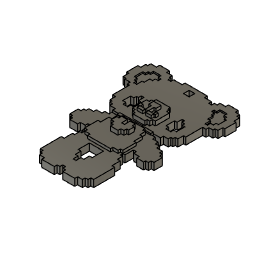
urs tema 1 varianta finala (Autodesk Fusion 360 design; units mm, degrees)
Autodesk Fusion 360 part; units mm, degrees
sketch "bear" plane through (0, 0, 0) normal (0, 0, 1) x (1, 0, 0)
  line L0 (-14, 45) -> (-7, 45)
  line L1 (-7, 45) -> (-7, 43)
  line L2 (-7, 43) -> (-3, 43)
  line L3 (-3, 43) -> (-3, 41)
  line L4 (-3, 41) -> (-2, 41)
  line L5 (-2, 41) -> (-2, 39)
  line L6 (-2, 39) -> (0, 39)
  line L7 (0, 39) -> (0, 41)
  line L8 (0, 41) -> (6, 41)
  line L9 (6, 41) -> (6, 43)
  line L10 (6, 43) -> (22, 43)
  line L11 (22, 43) -> (22, 41)
  line L12 (22, 41) -> (27, 41)
  line L13 (27, 41) -> (27, 39)
  line L14 (27, 39) -> (29, 39)
  line L15 (29, 39) -> (29, 41)
  line L16 (29, 41) -> (31, 41)
  line L17 (31, 41) -> (31, 43)
  line L18 (35, 43) -> (35, 45)
  line L19 (35, 45) -> (42, 45)
  line L20 (42, 45) -> (42, 43)
  line L21 (31, 43) -> (35, 43)
  line L22 (45, 43) -> (42, 43)
  line L23 (45, 43) -> (45, 41)
  line L24 (45, 41) -> (47, 41)
  line L25 (47, 41) -> (47, 37)
  line L26 (47, 37) -> (48.4791, 37)
  line L27 (48.4791, 37) -> (48.4791, 29)
  line L28 (48.4791, 29) -> (47, 29)
  line L29 (47, 29) -> (47, 25.5234)
  line L30 (47, 25.5234) -> (45, 25.5234)
  line L31 (45, 25.5234) -> (45, 24)
  line L32 (45, 24) -> (42, 24)
  line L33 (42, 24) -> (42, 22)
  line L34 (42, 22) -> (39.6461, 22)
  line L35 (39.6461, 22) -> (39.6461, 10)
  line L36 (39.6461, 10) -> (38, 10)
  line L37 (38, 10) -> (38, 6)
  line L38 (38, 6) -> (36, 6)
  line L39 (36, 6) -> (36, 4.4339)
  line L40 (36, 4.4339) -> (34.4937, 4.4339)
  line L41 (34.4937, 4.4339) -> (34.4937, 2.6047)
  line L42 (34.4937, 2.6047) -> (31.118, 2.6047)
  line L43 (31.118, 2.6047) -> (31.118, 0.4845)
  line L44 (31.118, 0.4845) -> (26, 0.4845)
  line L45 (26, 0.4845) -> (26, -1)
  line L46 (26, -1) -> (29, -1)
  line L47 (29, -1) -> (29, -3)
  line L48 (29, -3) -> (33, -3)
  line L49 (33, -3) -> (33, -5)
  line L50 (33, -5) -> (36, -5)
  line L51 (36, -5) -> (36, -7)
  line L52 (36, -7) -> (40, -7)
  line L53 (40, -7) -> (40, -9)
  line L54 (40, -9) -> (42, -9)
  line L55 (42, -9) -> (42, -11)
  line L56 (42, -11) -> (44, -11)
  line L57 (44, -11) -> (44, -17)
  line L58 (44, -17) -> (42, -17)
  line L59 (42, -17) -> (42, -19)
  line L60 (42, -19) -> (40, -19)
  line L61 (40, -19) -> (40, -20.3801)
  line L62 (40, -20.3801) -> (35, -20.3801)
  line L63 (35, -20.3801) -> (35, -18.5424)
  line L64 (35, -18.5424) -> (31, -18.5424)
  line L65 (31, -18.5424) -> (31, -16.5965)
  line L66 (31, -16.5965) -> (29, -16.5965)
  line L67 (29, -16.5965) -> (29, -22.6503)
  line L68 (29, -22.6503) -> (27.3439, -22.6503)
  line L69 (27.3439, -22.6503) -> (27.3439, -24.2966)
  line L70 (27.3439, -24.2966) -> (29, -24.2966)
  line L71 (29, -24.2966) -> (29, -28)
  line L72 (29, -28) -> (31, -28)
  line L73 (31, -28) -> (31, -34)
  line L74 (31, -34) -> (33, -34)
  line L75 (33, -34) -> (33, -49)
  line L76 (33, -49) -> (31, -49)
  line L77 (31, -49) -> (31, -51)
  line L78 (31, -51) -> (29, -51)
  line L79 (29, -51) -> (29, -53)
  line L80 (29, -53) -> (25.5718, -53)
  line L81 (25.5718, -53) -> (25.5718, -55)
  line L82 (25.5718, -55) -> (17, -55)
  line L83 (17, -55) -> (17, -53)
  line L84 (17, -53) -> (15, -53)
  line L85 (15, -53) -> (15, -51)
  line L86 (13, -51) -> (13, -53)
  line L87 (13, -53) -> (11, -53)
  line L88 (11, -53) -> (11, -55)
  line L89 (11, -55) -> (2, -55)
  line L90 (2, -55) -> (2, -53)
  line L91 (2, -53) -> (-1.5352, -53)
  line L92 (-1.5352, -53) -> (-1.5352, -51)
  line L93 (-1.5352, -51) -> (-3, -51)
  line L94 (-3, -51) -> (-3, -49)
  line L95 (-3, -49) -> (-5, -49)
  line L96 (-5, -49) -> (-5, -34)
  line L97 (-5, -34) -> (-3, -34)
  line L98 (-3, -34) -> (-3, -28)
  line L99 (-3, -28) -> (-1.486, -28)
  line L100 (-1.486, -28) -> (-1.486, -24.3526)
  line L101 (-1.486, -24.3526) -> (0, -24.3526)
  line L102 (0, -24.3526) -> (0, -22.7233)
  line L103 (0, -22.7233) -> (-1.486, -22.7233)
  line L104 (-1.486, -22.7233) -> (-1.486, -16.5263)
  line L105 (-1.486, -16.5263) -> (-3.4733, -16.5263)
  line L106 (-3.4733, -16.5263) -> (-3.4733, -18.4756)
  line L107 (-3.4733, -18.4756) -> (-7, -18.4756)
  line L108 (-7, -18.4756) -> (-7, -20.4249)
  line L109 (-7, -20.4249) -> (-12.5396, -20.4249)
  line L110 (-12.5396, -20.4249) -> (-12.5396, -18.4756)
  line L111 (-12.5396, -18.4756) -> (-14, -18.4756)
  line L112 (-14, -18.4756) -> (-14, -17)
  line L113 (-14, -17) -> (-16, -17)
  line L114 (-16, -17) -> (-16, -11)
  line L115 (-16, -11) -> (-14, -11)
  line L116 (-14, -11) -> (-14, -9)
  line L117 (-14, -9) -> (-12.403, -9)
  line L118 (-12.403, -9) -> (-12.403, -7)
  line L119 (-12.403, -7) -> (-9, -7)
  line L120 (-9, -7) -> (-9, -5)
  line L121 (-9, -5) -> (-5, -5)
  line L122 (-5, -5) -> (-5, -3)
  line L123 (-5, -3) -> (-2, -3)
  line L124 (-2, -3) -> (-2, -1)
  line L125 (-2, -1) -> (2, -1)
  line L126 (2, -1) -> (2, 0.5618)
  line L127 (2, 0.5618) -> (-3, 0.5618)
  line L128 (-3, 0.5618) -> (-3, 2.5032)
  line L129 (-3, 2.5032) -> (-7.0312, 2.5032)
  line L130 (-7.0312, 2.5032) -> (-7.0312, 4.4654)
  line L131 (-7.0312, 4.4654) -> (-9, 4.4654)
  line L132 (-9, 4.4654) -> (-9, 6)
  line L133 (-9, 6) -> (-10.3758, 6)
  line L134 (-10.3758, 6) -> (-10.3758, 10)
  line L135 (-10.3758, 10) -> (-12.4717, 10)
  line L136 (-12.4717, 10) -> (-12.4717, 22)
  line L137 (-12.4717, 22) -> (-14, 22)
  line L138 (-14, 22) -> (-14, 24)
  line L139 (-14, 24) -> (-18, 24)
  line L140 (-18, 24) -> (-18, 25)
  line L141 (-18, 25) -> (-20, 25)
  line L142 (-20, 25) -> (-20, 29)
  line L143 (-20, 29) -> (-21.5209, 29)
  line L144 (-21.5209, 29) -> (-21.5209, 37)
  line L145 (-21.5209, 37) -> (-19.4284, 37)
  line L146 (-19.4284, 37) -> (-19.4284, 40.542)
  line L147 (-19.4284, 40.542) -> (-18, 40.542)
  line L148 (-18, 40.542) -> (-18, 42.7271)
  line L149 (-18, 42.7271) -> (-14, 42.7271)
  line L150 (-14, 42.7271) -> (-14, 45)
  line L151 (15, -51) -> (14, -51)
  line L152 (14, -51) -> (14, -43.4733)
  line L153 (15, -43.4733) -> (15, -40)
  line L154 (15, -40) -> (17, -40)
  line L155 (17, -40) -> (17, -36)
  line L156 (17, -36) -> (19, -36)
  line L157 (19, -36) -> (19, -28)
  line L158 (19, -28) -> (9, -28)
  line L159 (9, -28) -> (9, -36)
  line L160 (9, -36) -> (11, -36)
  line L161 (11, -36) -> (11, -40)
  line L162 (11, -40) -> (13, -40)
  line L163 (13, -40) -> (13, -43.5179)
  line L164 (13, -51) -> (14, -51)
  line L165 (13, -43.5179) -> (14, -43.4733)
  line L166 (15, -43.4733) -> (14, -43.4733)
  line L167 (9, -5) -> (9, -7)
  line L168 (9, -7) -> (7.3877, -7)
  line L169 (7.3877, -7) -> (7.3877, -11)
  line L170 (7.3877, -11) -> (9.335, -11)
  line L171 (9.335, -11) -> (9.335, -13)
  line L172 (9.335, -13) -> (11, -13)
  line L173 (11, -13) -> (11, -15)
  line L174 (11, -15) -> (16.4316, -15)
  line L175 (16.4316, -15) -> (16.4316, -13)
  line L176 (16.4316, -13) -> (18.5952, -13)
  line L177 (18.5952, -13) -> (18.5952, -11)
  line L178 (18.5952, -11) -> (20, -11)
  line L179 (20, -11) -> (20, -7)
  line L180 (20, -7) -> (18.5952, -7)
  line L181 (18.5952, -7) -> (18.5952, -5)
  line L182 (18.5952, -5) -> (15, -5)
  line L183 (15, -5) -> (15, -7)
  line L184 (15, -7) -> (15, -9)
  line L185 (15, -9) -> (13, -9)
  line L186 (13, -9) -> (13, -7)
  line L187 (13, -7) -> (13, -5)
  line L188 (13, -5) -> (9, -5)
  line L189 (29.0368, 19.5758) -> (27.4228, 19.5758)
  line L190 (27.4228, 19.5758) -> (27.4228, 16)
  line L191 (27.4228, 16) -> (25.6136, 16)
  line L192 (25.6136, 16) -> (25.6136, 10)
  line L193 (25.6136, 10) -> (27.4228, 10)
  line L194 (27.4228, 10) -> (27.4228, 8)
  line L195 (27.4228, 8) -> (31, 8)
  line L196 (31, 8) -> (31, 10)
  line L197 (31, 10) -> (33, 10)
  line L198 (33, 10) -> (33, 16)
  line L199 (33, 16) -> (31, 16)
  line L200 (31, 16) -> (31, 17.6991)
  line L201 (31, 17.6991) -> (29.0368, 17.6991)
  line L202 (29.0368, 17.6991) -> (29.0368, 19.5758)
  line L203 (-1.6244, 19.559) -> (-1.6244, 17.5769)
  line L204 (-1.6244, 17.5769) -> (-3, 17.5769)
  line L205 (-3, 17.5769) -> (-3, 15.6458)
  line L206 (-3, 15.6458) -> (-5.3027, 15.6458)
  line L207 (-5.3027, 15.6458) -> (-5.3027, 10)
  line L208 (-5.3027, 10) -> (-3, 10)
  line L209 (-3, 10) -> (-3, 8)
  line L210 (-3, 8) -> (0.276, 8)
  line L211 (0.276, 8) -> (0.276, 10)
  line L212 (0.276, 10) -> (2, 10)
  line L213 (2, 10) -> (2, 15.6458)
  line L214 (2, 15.6458) -> (0.276, 15.6458)
  line L215 (0.276, 15.6458) -> (0.276, 19.559)
  line L216 (0.276, 19.559) -> (-1.6244, 19.559)
  line L217 (8.9896, 19.5636) -> (19, 19.5636)
  line L218 (19, 19.5636) -> (19, 18)
  line L219 (19, 18) -> (20, 18)
  line L220 (20, 18) -> (20, 16)
  line L221 (20, 16) -> (22, 16)
  line L222 (22, 16) -> (22, 6)
  line L223 (22, 6) -> (20, 6)
  line L224 (20, 6) -> (20, 4)
  line L225 (20, 4) -> (19, 4)
  line L226 (19, 4) -> (18, 4)
  line L227 (18, 4) -> (18, 2.4642)
  line L228 (18, 2.4642) -> (9.4555, 2.4642)
  line L229 (9.4555, 2.4642) -> (9.4555, 4)
  line L230 (9.4555, 4) -> (7.5988, 4)
  line L231 (7.5988, 4) -> (7.5988, 6)
  line L232 (7.5988, 6) -> (5.6945, 6)
  line L233 (5.6945, 6) -> (5.6945, 16)
  line L234 (5.6945, 16) -> (7.5988, 16)
  line L235 (7.5988, 16) -> (7.5988, 17.676)
  line L236 (7.5988, 17.676) -> (9, 17.676)
  line L237 (9, 17.676) -> (8.9896, 19.5636)
  line L238 (16.384, 15.6246) -> (16.384, 12)
  line L239 (16.384, 12) -> (15, 12)
  line L240 (15, 12) -> (15, 8)
  line L241 (15, 8) -> (18.5099, 8)
  line L242 (18.5099, 8) -> (18.5099, 10)
  line L243 (18.5099, 10) -> (20, 10)
  line L244 (20, 10) -> (20, 8)
  line L245 (20, 8) -> (19, 8)
  line L246 (19, 8) -> (19, 6)
  line L247 (19, 6) -> (15, 6)
  line L248 (15, 6) -> (15, 7.7223)
  line L249 (15, 7.7223) -> (13, 7.7223)
  line L250 (13, 7.7223) -> (13, 6)
  line L251 (13, 6) -> (9, 6)
  line L252 (9, 6) -> (9, 8)
  line L253 (9, 8) -> (7.4709, 8)
  line L254 (7.4709, 8) -> (7.4709, 10)
  line L255 (7.4709, 10) -> (9.3025, 10)
  line L256 (9.3025, 10) -> (9.3025, 8)
  line L257 (9.3025, 8) -> (13, 8)
  line L258 (13, 8) -> (13, 12.1247)
  line L259 (13, 12.1247) -> (11.1512, 12.1247)
  line L260 (11.1512, 12.1247) -> (11.1512, 15.6246)
  line L261 (11.1512, 15.6246) -> (16.384, 15.6246)
  line L262 (33.0271, 36.6906) -> (35, 36.6906)
  line L263 (35, 36.6906) -> (35, 39)
  line L264 (35, 39) -> (40, 39)
  line L265 (40, 39) -> (40, 36.6906)
  line L266 (40, 36.6906) -> (42, 36.6906)
  line L267 (42, 36.6906) -> (42, 35)
  line L268 (42, 35) -> (43.5849, 35)
  line L269 (43.5849, 35) -> (43.5849, 29.2707)
  line L270 (43.5849, 29.2707) -> (42, 29.2707)
  line L271 (42, 29.2707) -> (42, 27.2792)
  line L272 (42, 27.2792) -> (40, 27.2792)
  line L273 (40, 27.2792) -> (40, 25)
  line L274 (40, 25) -> (38.317, 25)
  line L275 (38.317, 25) -> (38.317, 29)
  line L276 (38.317, 29) -> (36.2934, 29)
  line L277 (36.2934, 29) -> (36.2934, 32.804)
  line L278 (36.2934, 32.804) -> (35, 32.804)
  line L279 (35, 32.804) -> (35, 35)
  line L280 (35, 35) -> (33.0271, 35)
  line L281 (33.0271, 35) -> (33.0271, 36.6906)
  line L282 (-5, 37) -> (-7, 37)
  line L283 (-7, 37) -> (-7, 39)
  line L284 (-7, 39) -> (-12.4235, 39)
  line L285 (-12.4235, 39) -> (-12.4235, 37)
  line L286 (-12.4235, 37) -> (-14, 37)
  line L287 (-14, 37) -> (-14, 35)
  line L288 (-14, 35) -> (-16, 35)
  line L289 (-16, 35) -> (-16, 29)
  line L290 (-16, 29) -> (-14, 29)
  line L291 (-14, 29) -> (-14, 27)
  line L292 (-14, 27) -> (-12.4235, 27)
  line L293 (-12.4235, 27) -> (-12.4235, 25)
  line L294 (-12.4235, 25) -> (-10.3514, 25)
  line L295 (-10.3514, 25) -> (-10.3514, 29)
  line L296 (-10.3514, 29) -> (-9, 29)
  line L297 (-9, 29) -> (-9, 33)
  line L298 (-9, 33) -> (-7, 33)
  line L299 (-7, 33) -> (-7, 35)
  line L300 (-7, 35) -> (-5, 35)
  line L301 (-5, 35) -> (-5, 37)
  line L302 (26, -1) -> (26, -1.349)
  line L303 (26, -1.349) -> (2, -1.349)
  line L304 (2, -1.349) -> (2, -1)
  line L305 (2, 0.5618) -> (26, 0.4845)
  line L306 (5.8111, -1.349) -> (5.8111, -3)
  line L307 (5.8111, -3) -> (4, -3)
  line L308 (4, -3) -> (4, -7)
  line L309 (4, -7) -> (2, -7)
  line L310 (2, -7) -> (2, -13)
  line L311 (2, -13) -> (0, -13)
  line L312 (0, -13) -> (0, -22.5439)
  line L313 (0, -22.5439) -> (2, -22.5439)
  line L314 (2, -22.5439) -> (2, -24.2549)
  line L315 (2, -24.2549) -> (5.662, -24.2549)
  line L316 (5.662, -24.2549) -> (5.662, -26)
  line L317 (5.662, -26) -> (22, -26)
  line L318 (22, -26) -> (22, -24.2549)
  line L319 (22, -24.2549) -> (25.7059, -24.2549)
  line L320 (25.7059, -24.2549) -> (25.7059, -22.5648)
  line L321 (25.7059, -22.5648) -> (27.352, -22.5648)
  line L322 (27.352, -22.5648) -> (27.352, -13)
  line L323 (27.352, -13) -> (25.7059, -13)
  line L324 (25.7059, -13) -> (25.7059, -7)
  line L325 (25.7059, -7) -> (23.853, -7)
  line L326 (23.853, -7) -> (23.853, -3)
  line L327 (23.853, -3) -> (22, -3)
  line L328 (22, -3) -> (22, -1.349)
  line L329 (-7, 33) -> (-9, 33)
  line L330 (12, 40) -> (16, 40)
  line L331 (16, 40) -> (16, 36)
  line L332 (16, 36) -> (12, 36)
  line L333 (12, 36) -> (12, 40)
  dimension "d21" = 16
  constraint horizontal L0
  constraint perpendicular L0 L1
  constraint perpendicular L1 L2
  constraint perpendicular L2 L3
  constraint perpendicular L3 L4
  constraint perpendicular L4 L5
  constraint perpendicular L5 L6
  constraint perpendicular L4 L7
  constraint perpendicular L7 L8
  constraint perpendicular L8 L9
  constraint perpendicular L9 L10
  constraint perpendicular L10 L11
  constraint perpendicular L9 L12
  constraint perpendicular L12 L13
  constraint perpendicular L9 L14
  constraint perpendicular L12 L15
  constraint perpendicular L15 L16
  constraint perpendicular L16 L17
  constraint perpendicular L16 L18
  constraint perpendicular L18 L19
  constraint perpendicular L19 L20
  constraint perpendicular L18 L21
  constraint perpendicular L20 L22
  constraint perpendicular L22 L23
  constraint perpendicular L20 L24
  constraint perpendicular L24 L25
  constraint perpendicular L23 L26
  constraint perpendicular L26 L27
  constraint perpendicular L27 L28
  constraint perpendicular L28 L29
  constraint perpendicular L29 L30
  constraint perpendicular L30 L31
  constraint perpendicular L31 L32
  constraint perpendicular L32 L33
  constraint perpendicular L33 L34
  constraint perpendicular L32 L35
  constraint perpendicular L33 L36
  constraint perpendicular L36 L37
  constraint perpendicular L37 L38
  constraint perpendicular L38 L39
  constraint perpendicular L39 L40
  constraint perpendicular L40 L41
  constraint perpendicular L41 L42
  constraint perpendicular L42 L43
  constraint perpendicular L43 L44
  constraint perpendicular L44 L45
  constraint perpendicular L45 L46
  constraint perpendicular L46 L47
  constraint perpendicular L45 L48
  constraint perpendicular L48 L49
  constraint perpendicular L49 L50
  constraint perpendicular L50 L51
  constraint perpendicular L49 L52
  constraint perpendicular L52 L53
  constraint perpendicular L49 L54
  constraint perpendicular L52 L55
  constraint perpendicular L55 L56
  constraint perpendicular L56 L57
  constraint perpendicular L57 L58
  constraint perpendicular L58 L59
  constraint perpendicular L59 L60
  constraint perpendicular L60 L61
  constraint perpendicular L59 L62
  constraint perpendicular L62 L63
  constraint perpendicular L59 L64
  constraint perpendicular L64 L65
  constraint perpendicular L65 L66
  constraint perpendicular L66 L67
  constraint perpendicular L67 L68
  constraint perpendicular L68 L69
  constraint perpendicular L69 L70
  constraint perpendicular L70 L71
  constraint perpendicular L71 L72
  constraint perpendicular L70 L73
  constraint perpendicular L71 L74
  constraint perpendicular L74 L75
  constraint perpendicular L75 L76
  constraint perpendicular L76 L77
  constraint perpendicular L77 L78
  constraint perpendicular L78 L79
  constraint perpendicular L79 L80
  constraint perpendicular L80 L81
  constraint perpendicular L81 L82
  constraint perpendicular L80 L83
  constraint perpendicular L81 L84
  constraint perpendicular L84 L85
  constraint perpendicular L86 L87
  constraint perpendicular L87 L88
  constraint perpendicular L86 L89
  constraint perpendicular L87 L90
  constraint perpendicular L90 L91
  constraint perpendicular L87 L92
  constraint perpendicular L92 L93
  constraint perpendicular L87 L94
  constraint perpendicular L92 L95
  constraint perpendicular L95 L96
  constraint perpendicular L92 L97
  constraint perpendicular L97 L98
  constraint perpendicular L98 L99
  constraint perpendicular L97 L100
  constraint perpendicular L100 L101
  constraint perpendicular L97 L102
  constraint perpendicular L100 L103
  constraint perpendicular L97 L104
  constraint perpendicular L104 L105
  constraint perpendicular L105 L106
  constraint perpendicular L106 L107
  constraint perpendicular L105 L108
  constraint perpendicular L108 L109
  constraint perpendicular L109 L110
  constraint perpendicular L110 L111
  constraint perpendicular L111 L112
  constraint perpendicular L110 L113
  constraint perpendicular L111 L114
  constraint perpendicular L114 L115
  constraint perpendicular L115 L116
  constraint perpendicular L116 L117
  constraint perpendicular L117 L118
  constraint perpendicular L118 L119
  constraint perpendicular L119 L120
  constraint perpendicular L120 L121
  constraint perpendicular L119 L122
  constraint perpendicular L122 L123
  constraint perpendicular L119 L124
  constraint perpendicular L122 L125
  constraint perpendicular L119 L126
  constraint perpendicular L126 L127
  constraint perpendicular L127 L128
  constraint perpendicular L126 L129
  constraint perpendicular L129 L130
  constraint perpendicular L130 L131
  constraint perpendicular L129 L132
  constraint perpendicular L132 L133
  constraint perpendicular L129 L134
  constraint perpendicular L134 L135
  constraint perpendicular L135 L136
  constraint perpendicular L136 L137
  constraint perpendicular L135 L138
  constraint perpendicular L138 L139
  constraint perpendicular L139 L140
  constraint perpendicular L138 L141
  constraint perpendicular L139 L142
  constraint perpendicular L142 L143
  constraint perpendicular L143 L144
  constraint perpendicular L144 L145
  constraint perpendicular L145 L146
  constraint perpendicular L146 L147
  constraint perpendicular L145 L148
  constraint perpendicular L146 L149
  constraint perpendicular L0 L150
  constraint perpendicular L85 L151
  constraint perpendicular L151 L152
  constraint perpendicular L152 L154
  constraint perpendicular L154 L155
  constraint perpendicular L155 L156
  constraint perpendicular L154 L157
  constraint perpendicular L155 L158
  constraint perpendicular L158 L159
  constraint perpendicular L155 L160
  constraint perpendicular L160 L161
  constraint perpendicular L161 L162
  constraint perpendicular L162 L163
  constraint perpendicular L152 L164
  constraint perpendicular L152 L166
  constraint vertical L167
  constraint perpendicular L167 L168
  constraint perpendicular L168 L169
  constraint perpendicular L169 L170
  constraint perpendicular L170 L171
  constraint perpendicular L169 L172
  constraint perpendicular L172 L173
  constraint perpendicular L169 L174
  constraint perpendicular L174 L175
  constraint perpendicular L175 L176
  constraint perpendicular L174 L177
  constraint perpendicular L177 L178
  constraint perpendicular L178 L179
  constraint perpendicular L177 L180
  constraint perpendicular L180 L181
  constraint perpendicular L177 L182
  constraint perpendicular L180 L183
  constraint perpendicular L180 L184
  constraint perpendicular L184 L185
  constraint perpendicular L185 L186
  constraint perpendicular L185 L187
  constraint perpendicular L167 L188
  constraint horizontal L189
  constraint perpendicular L189 L190
  constraint perpendicular L190 L191
  constraint perpendicular L189 L192
  constraint perpendicular L190 L193
  constraint perpendicular L193 L194
  constraint perpendicular L194 L195
  constraint perpendicular L193 L196
  constraint perpendicular L196 L197
  constraint perpendicular L197 L198
  constraint perpendicular L196 L199
  constraint perpendicular L199 L200
  constraint perpendicular L196 L201
  constraint perpendicular L201 L202
  constraint vertical L203
  constraint perpendicular L203 L204
  constraint perpendicular L204 L205
  constraint perpendicular L205 L206
  constraint perpendicular L206 L207
  constraint perpendicular L205 L208
  constraint perpendicular L206 L209
  constraint perpendicular L205 L210
  constraint perpendicular L206 L211
  constraint perpendicular L211 L212
  constraint perpendicular L206 L213
  constraint perpendicular L211 L214
  constraint perpendicular L206 L215
  constraint perpendicular L203 L216
  constraint horizontal L217
  constraint perpendicular L217 L218
  constraint perpendicular L218 L219
  constraint perpendicular L219 L220
  constraint perpendicular L220 L221
  constraint perpendicular L219 L222
  constraint perpendicular L222 L223
  constraint perpendicular L223 L224
  constraint perpendicular L224 L225
  constraint perpendicular L224 L226
  constraint perpendicular L226 L227
  constraint perpendicular L227 L228
  constraint perpendicular L228 L229
  constraint perpendicular L229 L230
  constraint perpendicular L228 L231
  constraint perpendicular L229 L232
  constraint perpendicular L232 L233
  constraint perpendicular L233 L234
  constraint perpendicular L234 L235
  constraint perpendicular L235 L236
  constraint perpendicular L217 L238
  constraint perpendicular L238 L239
  constraint perpendicular L239 L240
  constraint perpendicular L238 L241
  constraint perpendicular L241 L242
  constraint perpendicular L242 L243
  constraint perpendicular L243 L244
  constraint perpendicular L242 L245
  constraint perpendicular L245 L246
  constraint perpendicular L246 L247
  constraint perpendicular L247 L248
  constraint perpendicular L246 L249
  constraint perpendicular L249 L250
  constraint perpendicular L250 L251
  constraint perpendicular L251 L252
  constraint perpendicular L252 L253
  constraint perpendicular L253 L254
  constraint perpendicular L254 L255
  constraint perpendicular L255 L256
  constraint perpendicular L254 L257
  constraint perpendicular L255 L258
  constraint perpendicular L254 L259
  constraint perpendicular L259 L260
  constraint perpendicular L260 L261
  constraint horizontal L262
  constraint perpendicular L262 L263
  constraint perpendicular L263 L264
  constraint perpendicular L264 L265
  constraint perpendicular L263 L266
  constraint perpendicular L266 L267
  constraint perpendicular L267 L268
  constraint perpendicular L268 L269
  constraint perpendicular L269 L270
  constraint perpendicular L270 L271
  constraint perpendicular L271 L272
  constraint perpendicular L272 L273
  constraint perpendicular L273 L274
  constraint perpendicular L274 L275
  constraint perpendicular L273 L276
  constraint perpendicular L274 L277
  constraint perpendicular L273 L278
  constraint perpendicular L274 L279
  constraint perpendicular L273 L280
  constraint perpendicular L280 L281
  constraint perpendicular L144 L282
  constraint perpendicular L282 L283
  constraint perpendicular L144 L284
  constraint perpendicular L284 L285
  constraint perpendicular L285 L286
  constraint perpendicular L284 L287
  constraint perpendicular L287 L288
  constraint perpendicular L284 L289
  constraint perpendicular L287 L290
  constraint perpendicular L290 L291
  constraint perpendicular L287 L292
  constraint perpendicular L292 L293
  constraint perpendicular L287 L294
  constraint perpendicular L292 L295
  constraint perpendicular L295 L296
  constraint perpendicular L292 L297
  constraint perpendicular L297 L298
  constraint perpendicular L292 L299
  constraint perpendicular L299 L300
  constraint perpendicular L282 L301
  constraint perpendicular L46 L302
  constraint perpendicular L126 L303
  constraint perpendicular L125 L304
  constraint coincident L303 L306.start
  constraint perpendicular L303 L306
  constraint perpendicular L306 L307
  constraint perpendicular L303 L308
  constraint perpendicular L308 L309
  constraint perpendicular L303 L310
  constraint perpendicular L310 L311
  constraint perpendicular L311 L312
  constraint perpendicular L312 L313
  constraint perpendicular L311 L314
  constraint perpendicular L314 L315
  constraint perpendicular L315 L316
  constraint perpendicular L314 L317
  constraint perpendicular L317 L318
  constraint perpendicular L318 L319
  constraint perpendicular L319 L320
  constraint perpendicular L320 L321
  constraint perpendicular L319 L322
  constraint perpendicular L320 L323
  constraint perpendicular L323 L324
  constraint perpendicular L320 L325
  constraint perpendicular L323 L326
  constraint perpendicular L320 L327
  constraint coincident L303 L328.end
  constraint perpendicular L303 L328
  constraint perpendicular L9 L330
  constraint perpendicular L330 L331
  constraint perpendicular L331 L332
  constraint perpendicular L330 L333
  measures "d21" distance of L9.end L10.end
extrude "Extrude1" add sketch "bear" along normal blind 5 contours L0 L1 L2 L3 L4 L5 L6 L7 L8 L9 L10 L11 L12 L13 L14 L15 L16 L17 L18 L19 L20 L21 L22 L23 L24 L25 L26 L27 L28 L29 L30 L31 L32 L33 L34 L35 L36 L37 L38 L39 L40 L41 L42 L43 L44 L127 L128 L129 L130 L131 L132 L133 L134 L135 L136 L137 L138 L139 L140 L141 L142 L143 L144 L145 L146 L147 L148 L149 L150 L305 | L46 L47 L48 L49 L50 L51 L52 L53 L54 L55 L56 L57 L58 L59 L60 L61 L62 L63 L64 L65 L66 L67 L68 L69 L70 L71 L72 L73 L74 L75 L76 L77 L78 L79 L80 L81 L82 L83 L84 L85 L86 L87 L88 L89 L90 L91 L92 L93 L94 L95 L96 L97 L98 L99 L100 L101 L102 L103 L104 L105 L106 L107 L108 L109 L110 L111 L112 L113 L114 L115 L116 L117 L118 L119 L120 L121 L122 L123 L124 L125 L151 L164 L302 L303 L304 L306 L307 L308 L309 L310 L311 L312 L313 L314 L315 L316 L317 L318 L319 L320 L321 L322 L323 L324 L325 L326 L327 L328 makes body 1 at (4.092, 31.5197, 0) makes body 2 at (1, -39.6667, 0)
extrude "Extrude2" add sketch "bear" along normal blind 8 separate body contours L217 L218 L219 L220 L221 L222 L223 L224 L225 L226 L227 L228 L229 L230 L231 L232 L233 L234 L235 L236 L237 makes body 3
extrude "Extrude3" add sketch "bear" along normal blind 10 separate body contours L238 L239 L240 L241 L242 L243 L244 L245 L246 L247 L248 L249 L250 L251 L252 L253 L254 L255 L256 L257 L258 L259 L260 L261 makes body 4
extrude "Extrude4" add sketch "bear" along normal blind 7 separate body contours L303 L306 L307 L308 L309 L310 L311 L312 L313 L314 L315 L316 L317 L318 L319 L320 L321 L322 L323 L324 L325 L326 L327 L328 makes body 5
extrude "Extrude5" add sketch "bear" along normal blind 10 separate body contours L167 L168 L169 L170 L171 L172 L173 L174 L175 L176 L177 L178 L179 L180 L181 L182 L183 L184 L185 L186 L187 L188 makes body 6
extrude "Extrude6" add sketch "bear" along normal blind 4 separate body contours L262 L263 L264 L265 L266 L267 L268 L269 L270 L271 L272 L273 L274 L275 L276 L277 L278 L279 L280 L281 | L282 L283 L284 L285 L286 L287 L288 L289 L290 L291 L292 L293 L294 L295 L296 L297 L298 L299 L300 L301 L329 makes body 7 at (38.8701, 32.268, 0) makes body 8 at (-12.3333, 32.3333, 0)
extrude "Extrude7" add sketch "bear" along normal blind 6 contours L45 L126 L302 L303 L304 L305 bodies 2 3 4 6 7 8 1 5
combine "Combine1" operation add target body 2 tool bodies 3 4 6 7 8
named bodies: "bear ok"
